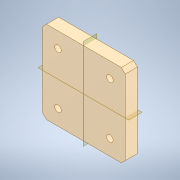
# Autodesk Inventor part: Front Armor
Saved by Autodesk Inventor 2022 (Build 260153000, 153)
## iProperties
Created: 2022-08-21
Part Number: Front Armor
Material: Polyethylene, High Density
Document SubType Name: Modeling
Designer: Nick
Density: 0.952 g/cm^3
Appearance: Smooth - Off-White
Mass: 10.9097 g
Surface Area: 49.4312 cm^2
Volume: 11.4597 cm^3
Author: Nick
Autodesk Inventor part; units mm, degrees
ref_plane "YZ Plane" through (0, 0, 0) normal (1, 0, 0) x (0, 1, 0)
ref_plane "XZ Plane" through (0, 0, 0) normal (0, 1, 0) x (-1, 0, 0)
ref_plane "XY Plane" through (0, 0, 0) normal (0, 0, 1) x (1, 0, 0)
sketch "Sketch1" plane through (0, 0, 0) normal (0, 0, 1) x (1, 0, 0)
  line L0 (0, 0) -> (43, 0)
  line L1 (43, 0) -> (43, 43)
  line L2 (43, 43) -> (0, 43)
  line L3 (0, 43) -> (0, 0)
  dimension "d0" = 43
  dimension "d1" = 43
  constraints: 8 end point, 2 parallel, 1 horizontal, 1 perpendicular
  measures "d0" distance of L2.end L1.end
  measures "d1" distance of L1.end L0.end
extrude "Extrusion1" add sketch "Sketch1" along normal blind 6.35
chamfer "Chamfer1" distance 2 angle 45 4 edges at (43, 43, 3.175) (43, 0, 3.175) (0, 43, 3.175) (0, 0, 3.175)
sketch "Sketch2" plane through (0, 0, 6.35) normal (0, 0, 1) x (1, 0, 0)
  line L0 (0, 41) -> (0, 2) projected
  line L1 (43, 2) -> (43, 41) projected
  line L2 (2, 0) -> (41, 0) projected
  line L3 (41, 43) -> (2, 43) projected
  point P0 (0, 0)
  point P1 (8, 8)
  point P2 (35, 8)
  point P3 (35, 35)
  point P4 (8, 35)
  dimension "d7" = 8
  dimension "d8" = 8
  dimension "d9" = 8
  dimension "d10" = 8
  dimension "d11" = 8
  dimension "d12" = 8
  constraints: 2 horizontal alignment
  measures "d7" distance from line of L0 point (8, 8)
  measures "d8" distance from line of L1 point (35, 8)
  measures "d9" distance from line of L2 point (35, 8)
  measures "d10" distance from line of L3 point (35, 35)
  measures "d11" distance from line of L1 point (35, 35)
  measures "d12" distance from line of L0 point (8, 35)
hole "Hole1" at (8, 8, 6.35) at (35, 8, 6.35) at (35, 35, 6.35) at (8, 35, 6.35) direction (0, 0, -1) diameter 3.4 depth 7 tip angle 118 clearance for "Flat Head Machine Screw" size "M3" standard "Ansi Metric M Profile"
ref_plane "Work Plane1" through (2, 21.5, 0) normal (0, 1, 0) x (1, 0, 0)
ref_plane "Work Plane2" through (21.5, 2, 0) normal (-1, 0, 0) x (0, 0, 1)
body "Solid1"
